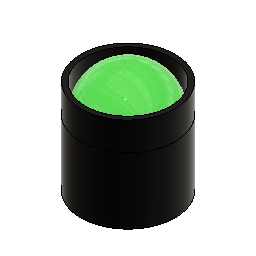
TETRA V7 (Autodesk Fusion 360 archive; units mm, degrees)
design "Palm Beach Bots Antweight Light & Mount"
part number: 2026-04-12-16-16-46-918
Autodesk Fusion 360 part; units mm, degrees
sketch "Sketch1" plane through (0, 0, 0) normal (0, 1, 0) x (1, 0, 0)
  circle A0 centre (0, 0) radius 2.5
  constraint coincident A0.centre origin
extrude "Extrude1" add sketch "Sketch1" along normal blind 3.5 makes body 1
sphere "SpherePrimitive1" add diameter 4.5 placed x (-1, 0, 0) y (0, 0, 1) z (0, 1, 0) at (0, 3.5, 0) separate body makes body 2
sketch "Sketch3" plane through (0, 0, 0) normal (0, 1, 0) x (1, 0, 0)
  circle A0 centre (0, 0) radius 2.5
  circle A1 centre (0, 0) radius 2.25
  dimension "d4" = 4.5
  constraint coincident A0.centre A1.centre
  constraint concentric A0 A1
  measures "d4" diameter of A1
extrude "Extrude2" add sketch "Sketch3" along normal blind 5 separate body makes body 3

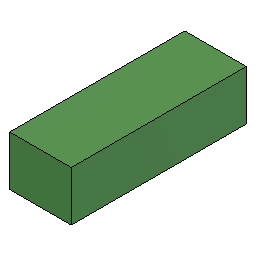
design "Palm Power Gen2 2S 300mAh 7.4v 65c LiPo Battery"
part number: 2026-04-12-16-28-50-413
Autodesk Fusion 360 part; units mm, degrees
sketch "Sketch1" plane through (0, 0, 0) normal (0, 1, 0) x (1, 0, 0)
  line L0 (0, 0) -> (16.25, 0)
  line L1 (16.25, 0) -> (16.25, 46.2)
  line L2 (16.25, 46.2) -> (0, 46.2)
  line L3 (0, 46.2) -> (0, 0)
  dimension "d1" = 16.25
  dimension "d2" = 46.2
  constraint horizontal L0
  constraint vertical L1
  constraint horizontal L2
  constraint vertical L3
  constraint coincident L0.start L3.end
  measures "d1" distance of L0.start L0.end
  measures "d2" distance of L0.start L2.end
extrude "Extrude1" add sketch "Sketch1" along normal blind 13.15
